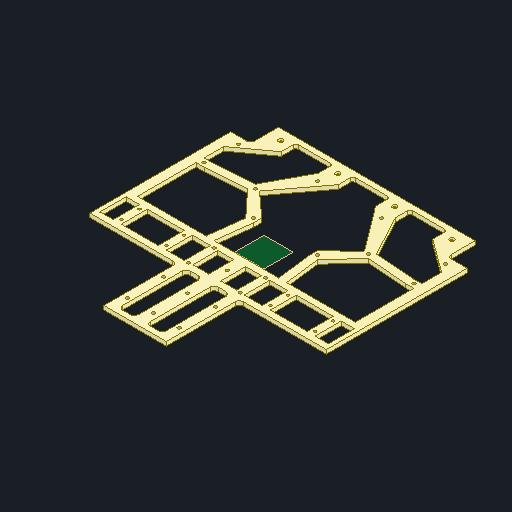
# Autodesk Inventor part: base
Saved by Autodesk Inventor 2023 (Build 270158000, 158)
## iProperties
Created: 2024-04-10
Part Number: base
Material: Nylon 6/6
Document SubType Name: Modeling
Designer: szymo
Density: 1.13 g/cm^3
Appearance: Nylon 6
Mass: 28.9572 g
Surface Area: 254.405 cm^2
Volume: 25.6258 cm^3
Author: szymo
Autodesk Inventor part; units mm, degrees
ref_plane "YZ Plane" through (0, 0, 0) normal (1, 0, 0) x (0, 1, 0)
ref_plane "XZ Plane" through (0, 0, 0) normal (0, 1, 0) x (-1, 0, 0)
ref_plane "XY Plane" through (0, 0, 0) normal (0, 0, 1) x (1, 0, 0)
sketch "Sketch2" plane through (0, 0, 0) normal (0, 1, 0) x (-1, 0, 0)
  line L0 (-89, 99) -> (89, 99)
  line L1 (89, 99) -> (89, -99)
  line L2 (89, -99) -> (-89, -99)
  line L3 (-89, -99) -> (-89, 99)
  line L4 (-89, 99) -> (89, -99) construction
  line L5 (89, 99) -> (-89, -99) construction
  line L6 (-89, 99) -> (89, 99)
  line L7 (89, 99) -> (89, -85)
  line L8 (89, -85) -> (-89, -85)
  line L9 (-89, -85) -> (-89, 99)
  line L10 (-4.5, 99) -> (-89, 99)
  line L11 (-89, 99) -> (-89, 42)
  line L12 (-89, 42) -> (-4.5, 42)
  line L13 (-4.5, 42) -> (-4.5, 99)
  line L14 (4.5, 99) -> (89, 99)
  line L15 (89, 99) -> (89, 42)
  line L16 (89, 42) -> (4.5, 42)
  line L17 (4.5, 42) -> (4.5, 99)
  line L18 (22.5, 77.5) -> (22.5, 66.5) projected
  line L19 (16.5, 66.5) -> (16.5, 77.5) projected
  line L20 (-22.5, 66.5) -> (-22.5, 77.5) projected
  line L21 (-16.5, 77.5) -> (-16.5, 66.5) projected
  line L22 (-23.5, 99) -> (-16.5, 99)
  line L23 (-16.5, 99) -> (-16.5, 42)
  line L24 (-16.5, 42) -> (-23.5, 42)
  line L25 (-23.5, 42) -> (-23.5, 99)
  line L26 (16.5, 99) -> (23.5, 99)
  line L27 (23.5, 99) -> (23.5, 42)
  line L28 (23.5, 42) -> (16.5, 42)
  line L29 (16.5, 42) -> (16.5, 99)
  line L30 (-89, 99) -> (89, 99)
  line L31 (89, 99) -> (89, 97)
  line L32 (89, 97) -> (-89, 97)
  line L33 (-89, 97) -> (-89, 99)
  line L34 (89, -85) -> (74, -85)
  line L35 (74, -85) -> (74, -64)
  line L36 (74, -64) -> (89, -64)
  line L37 (89, -64) -> (89, -85)
  line L38 (-89, -85) -> (-74, -85)
  line L39 (-74, -85) -> (-74, -64)
  line L40 (-74, -64) -> (-89, -64)
  line L41 (-89, -64) -> (-89, -85)
  line L42 (16.5, 97) -> (-16.5, 97)
  line L43 (-16.5, 97) -> (-16.5, 93)
  line L44 (-16.5, 93) -> (16.5, 93)
  line L45 (16.5, 93) -> (16.5, 97)
  line L46 (-84.4, -75) -> (-84.4, -71.5) projected
  line L47 (-84.4, -71.5) -> (-87, -71.5) projected
  line L48 (-87, -71.5) -> (-87, -75) projected
  line L49 (-87, -75) -> (-84.4, -75) projected
  line L50 (-79.6, -75) -> (-77, -75) projected
  line L51 (-77, -75) -> (-77, -71.5) projected
  line L52 (-77, -71.5) -> (-79.6, -71.5) projected
  line L53 (-79.6, -71.5) -> (-79.6, -75) projected
  line L54 (-75, -78) -> (-89, -78) projected
  line L55 (-89, -78) -> (-89, -63) projected
  line L56 (-89, -63) -> (-75, -63) projected
  line L57 (-75, -63) -> (-75, -78) projected
  circle A0 centre (-80.45, -67.25) radius 1.25 projected
  point P0 (0, 0)
  point P1 (4.5, 99)
  point P2 (-4.5, 99)
  point P3 (-89, 42)
  point P4 (89, 42)
  point P5 (4.5, 97)
  point P6 (-4.5, 97)
  point P7 (-16.5, 97)
  point P8 (-23.5, 97)
  point P9 (23.5, 97)
  point P10 (16.5, 98)
  point P11 (-4.5, 93)
  point P12 (4.5, 93)
  point P13 (16.5, 93)
  dimension "d8" = 178
  dimension "d9" = 198
  dimension "d10" = 14
  dimension "d11" = 84.5
  dimension "d13" = 84.5
  dimension "d17" = 9
  dimension "d18" = 2
  dimension "d19" = 15
  dimension "d20" = 21
  dimension "d21" = 15
  dimension "d22" = 21
  dimension "d75" = 55
  dimension "d76" = 55
  dimension "d77" = 7
  dimension "d78" = 7
  dimension "d79" = 4
  constraints: 84 end point, 20 parallel, 10 horizontal, 10 perpendicular, 10 point on line, 2 collinear, 2 midpoint, 5 other
  measures "d8" distance of L1.end L2.end
  measures "d9" distance of L0.end L1.end
  measures "d10" distance between parallel lines of L8 L2
  measures "d11" distance of L12.end L11.end
  measures "d13" distance of L15.end L16.end
  measures "d17" distance between parallel lines of L13 L17
  measures "d18" distance of L30.end L31.end
  measures "d19" distance of L35.end L36.end
  measures "d20" distance of L34.end L35.end
  measures "d21" distance of L40.end L39.end
  measures "d22" distance of L39.end L38.end
  measures "d75" distance between parallel lines of L32 L12
  measures "d76" distance between parallel lines of L32 L16
  measures "d77" distance between parallel lines of L23 L25
  measures "d78" distance between parallel lines of L27 L29
  measures "d79" distance of L43.end L42.end
extrude "Extrusion2" add sketch "Sketch2" along normal blind 3 contours L32 L23 L21 L12 L25 | L12 L13 L44 L17 L16 L1 L36 L35 L8 L39 L40 L57 L56 L3 | L32 L13 L44 L23 | L56 L57 L40 L3 | L32 L17 L44 L13 | L32 L29 L44 L17 | L32 L27 L16 L29 L19
fillet "Fillet5" radius 3 12 edges at (-16.5, 1.5, 42) (-4.5, 1.5, 42) (-23.5, 1.5, 42) (16.5, 1.5, 42) (-16.5, 1.5, 93) (-4.5, 1.5, 93) (4.5, 1.5, 93) (16.5, 1.5, 93) (4.5, 1.5, 42) (23.5, 1.5, 42) (74, 1.5, -64) (-74, 1.5, -64)
sketch "Sketch7" plane through (0, 3, 0) normal (0, 1, 0) x (1, 0, 0)
  circle A0 centre (78, 58.6725) radius 1.8 projected
  circle A1 centre (79, 33.8889) radius 1.8 projected
  circle A2 centre (42.4984, 36.1666) radius 1.8 projected
  circle A3 centre (24.1, 64.6) radius 1.6 projected
  circle A4 centre (24.1, 16.4) radius 1.6 projected
  circle A5 centre (-24.1, 16.4) radius 1.6 projected
  circle A6 centre (-24.1, 64.6) radius 1.6 projected
  circle A7 centre (-42.5, 36.1649) radius 1.8 projected
  circle A8 centre (-79, 33.8889) radius 1.8 projected
  circle A9 centre (-78, 58.6725) radius 1.8 projected
  circle A10 centre (19.5, -18.05) radius 1.8 projected
  circle A11 centre (19.5, -37.375) radius 1.8 projected
  circle A12 centre (19.5, -55.8) radius 1.8 projected
  circle A13 centre (19.4231, -83.3077) radius 1.8 projected
  circle A14 centre (0, -83.2) radius 1.8 projected
  circle A15 centre (-19.4231, -83.3077) radius 1.8 projected
  circle A16 centre (-19.5, -55.8) radius 1.8 projected
  circle A17 centre (0, -57.55) radius 1.8 projected
  circle A18 centre (0, -27.625) radius 1.8 projected
  circle A19 centre (-19.5, -37.375) radius 1.8 projected
  circle A20 centre (-19.5, -18.05) radius 1.8 projected
  point P0 (0, 0)
  point P1 (-19.5, -83.2)
  constraints: 20 coincident
hole "Hole3" at (19.4231, 3, 83.3077) at (0, 3, 83.2) at (-19.5, 3, 83.2) at (19.5, 3, 55.8) at (0, 3, 57.55) at (-19.5, 3, 55.8) at (-19.5, 3, 37.375) at (-19.5, 3, 18.05) at (0, 3, 27.625) at (19.5, 3, 37.375) at (19.5, 3, 18.05) at (79, 3, -33.8889) at (78, 3, -58.6725) at (42.4984, 3, -36.1666) at (24.1, 3, -16.4) at (-24.1, 3, -16.4) at (-24.1, 3, -64.6) at (24.1, 3, -64.6) at (-42.5, 3, -36.1649) at (-78, 3, -58.6725) at (-79, 3, -33.8889) direction (0, -1, 0) diameter 2.459 end through all thread size "M3x0.5" class "6H" standard "ISO Metric profile"
sketch "Sketch8" plane through (0, 3, 0) normal (0, 1, 0) x (1, 0, 0)
  circle A0 centre (86, 37.5556) radius 2.3 projected
  line L0 (89, 40.5556) -> (89, -42) projected
  line L1 (89, 40.5556) -> (83, 40.5556) projected
  line L2 (83, 34.5556) -> (87.4, 34.5556) projected
  line L3 (87.4, 34.5556) -> (87.4, 19.4556) projected
  line L4 (87.4, 19.4556) -> (86, 19.4556) projected
  line L5 (86, -36) -> (86, 19.4556) projected
  circle A1 centre (-86, -39) radius 2.3 projected
  circle A2 centre (-86, -16.25) radius 2.3 projected
  line L6 (-86, -13.25) -> (-86, 29.8889) projected
  line L7 (-86, -36) -> (-86, -19.25) projected
  line L8 (-86, 29.8889) -> (-83, 29.8889) projected
  line L9 (-83, 29.8889) -> (-83, 35.8889) projected
  line L10 (-89, 35.8889) -> (-83, 35.8889) projected
  line L11 (-89, 35.8889) -> (-89, -42) projected
  line L12 (-89, -42) -> (-83, -42) projected
  line L13 (-83, -42) -> (-83, -36) projected
  line L14 (-83, -36) -> (-86, -36) projected
  line L15 (-86, -19.25) -> (-83, -19.25) projected
  line L16 (-83, -19.25) -> (-83, -13.25) projected
  line L17 (-83, -13.25) -> (-86, -13.25) projected
  circle A3 centre (-86, 32.8889) radius 2.3 projected
  ellipse E0 centre (-72.9406, -34.421) end of major axis (-70.1906, -34.421) minor radius 2.75 projected
  ellipse E1 centre (-72.9594, -20.7569) end of major axis (-70.2094, -20.7569) minor radius 2.75 projected
  ellipse E2 centre (-39.125, -20.8137) end of major axis (-36.375, -20.8137) minor radius 2.75 projected
  ellipse E3 centre (-39.125, -34.3886) end of major axis (-36.375, -34.3886) minor radius 2.75 projected
  ellipse E4 centre (39.125, -20.8137) end of major axis (36.375, -20.8137) minor radius 2.75 projected
  ellipse E5 centre (39.125, -34.3886) end of major axis (36.375, -34.3886) minor radius 2.75 projected
  ellipse E6 centre (72.9406, -34.421) end of major axis (70.1906, -34.421) minor radius 2.75 projected
  ellipse E7 centre (72.9594, -20.7569) end of major axis (70.2094, -20.7569) minor radius 2.75 projected
  line L18 (89, -42) -> (83, -42) projected
  line L19 (83, 34.5556) -> (83, 40.5556) projected
  circle A4 centre (86, -39) radius 2.3 projected
  line L20 (86, -36) -> (83, -36) projected
  line L21 (83, -36) -> (83, -42) projected
  point P0 (0, 0)
  point P1 (83, 35.8889)
  point P2 (72.95, -34.475)
  point P3 (72.95, -20.775)
  point P4 (39.125, -20.8375)
  point P5 (39.125, -34.4125)
  point P6 (86, -39)
  point P7 (86, -16.25)
  point P8 (-72.95, -20.775)
  point P9 (-72.95, -34.475)
  point P10 (-39.125, -34.4125)
  point P11 (-39.125, -20.8375)
  constraints: 2 coincident, 4 other
hole "Hole4" at (72.95, 3, 34.475) at (72.95, 3, 20.775) at (39.125, 3, 20.8375) at (39.125, 3, 34.4125) at (-72.95, 3, 20.775) at (-72.95, 3, 34.475) at (-39.125, 3, 34.4125) at (-39.125, 3, 20.8375) direction (0, -1, 0) diameter 2.013 end through all thread size "M2.5x0.45" class "6H" standard "ISO Metric profile"
ref_plane "Work Plane1" through (0, 1, 0) normal (0, -1, 0) x (1, 0, 0)
sketch "Sketch13" plane through (0, 0, 0) normal (0, -1, 0) x (1, 0, 0)
  circle A0 centre (21.5, -77) radius 1.2295 projected
  circle A1 centre (-64.5, -77) radius 1.2295 projected
  circle A2 centre (-21.5, -77) radius 1.2295 projected
  circle A3 centre (64.5, -77) radius 1.2295 projected
  line L0 (-72, -79) -> (-72, -70) projected
  line L1 (-72, -70) -> (-57, -70) projected
  line L2 (-57, -70) -> (-57, -79) projected
  arc A4 (-57, -79) -> (-55, -81) centre (-55, -79) ccw projected
  line L3 (-55, -81) -> (-31, -81) projected
  arc A5 (-31, -81) -> (-29, -79) centre (-31, -79) ccw projected
  line L4 (-29, -79) -> (-29, -70) projected
  line L5 (-29, -70) -> (-14, -70) projected
  line L6 (-14, -70) -> (-14, -79) projected
  arc A6 (-14, -79) -> (-12, -81) centre (-12, -79) ccw projected
  line L7 (-12, -81) -> (12, -81) projected
  arc A7 (12, -81) -> (14, -79) centre (12, -79) ccw projected
  line L8 (14, -79) -> (14, -70) projected
  line L9 (14, -70) -> (29, -70) projected
  line L10 (29, -70) -> (29, -79) projected
  arc A8 (29, -79) -> (31, -81) centre (31, -79) ccw projected
  line L11 (31, -81) -> (55, -81) projected
  arc A9 (55, -81) -> (57, -79) centre (55, -79) ccw projected
  line L12 (57, -79) -> (57, -70) projected
  line L13 (57, -70) -> (72, -70) projected
  line L14 (72, -70) -> (72, -79) projected
  arc A10 (72, -79) -> (74, -81) centre (74, -79) ccw projected
  line L15 (74, -81) -> (89, -81) projected
  line L16 (89, -85) -> (89, -81) projected
  line L17 (-89, -85) -> (89, -85) projected
  line L18 (-89, -85) -> (-89, -81) projected
  line L19 (-89, -81) -> (-74, -81) projected
  arc A11 (-74, -81) -> (-72, -79) centre (-74, -79) ccw projected
  point P0 (0, 0)
  constraints: 4 coincident
hole "Hole6" at (64.5, 0, -77) at (21.5, 0, -77) at (-21.5, 0, -77) at (-64.5, 0, -77) direction (0, 1, 0) diameter 3.6 end through all countersink diameter 6.7 countersink angle 90 clearance for "Countersunk Flat Head Screw ISO 2009/7046" size "M3" standard "ISO"
ref_plane "Work Plane2" through (0, 1, 0) normal (0, -1, 0) x (1, 0, 0)
sketch "Sketch14" plane through (0, 0, 0) normal (0, -1, 0) x (1, 0, 0)
  circle A0 centre (-42.5, -36.1649) radius 1.8 projected
  line L0 (-86, -29.8889) -> (-86, 42) projected
  line L1 (-89, 42) -> (-86, 42) projected
  line L2 (-89, 42) -> (-89, 38.75) projected
  line L3 (-89, 38.75) -> (-89, 13.5) projected
  line L4 (-89, 13.5) -> (-89, -81) projected
  line L5 (-89, -81) -> (-83, -81) projected
  line L6 (-83, -81) -> (-83, -75) projected
  line L7 (-83, -75) -> (-73, -75) projected
  line L8 (-73, -75) -> (-73, -53.3451) projected
  line L9 (-73, -53.3451) -> (-67, -53.3451) projected
  line L10 (-67, -53.3451) -> (-67, -42.9318) projected
  line L11 (-76.801, -42.9318) -> (-67, -42.9318) projected
  ellipse E0 centre (-76.799, -27.2986) end of major axis (-76.7969, -11.6653) minor radius 1.851 (-77.5308, -41.6649) -> (-76.801, -42.9318) ccw projected
  line L12 (-46, -41.6649) -> (-77.5308, -41.6649) projected
  line L13 (-46, -39.6649) -> (-46, -41.6649) projected
  line L14 (-39, -39.6649) -> (-46, -39.6649) projected
  line L15 (-39, -32.6649) -> (-39, -39.6649) projected
  line L16 (-46, -32.6649) -> (-39, -32.6649) projected
  line L17 (-46, -29.8889) -> (-46, -32.6649) projected
  line L18 (-46, -29.8889) -> (-52, -29.8889) projected
  line L19 (-52, -34.8889) -> (-52, -29.8889) projected
  line L20 (-75, -34.8889) -> (-52, -34.8889) projected
  line L21 (-75, -34.8889) -> (-75, -29.8889) projected
  line L22 (-86, -29.8889) -> (-75, -29.8889) projected
  circle A1 centre (-83.5, -70.5) radius 1.75 projected
  circle A2 centre (-79, -33.8889) radius 1.8 projected
  circle A3 centre (-78, -58.6725) radius 1.8 projected
  circle A4 centre (78, -58.6725) radius 1.8 projected
  circle A5 centre (79, -33.8889) radius 1.8 projected
  circle A6 centre (80.5, -70.5) radius 1.75 projected
  circle A7 centre (42.4984, -36.1666) radius 1.8 projected
  spline S0 degree 2 poles (89, 38.051) (88.5208, 39.25) (89, 40.449) knots 0 0 0 0.244949 0.244949 0.244949 weights 1 1.090909 1 projected
  line L23 (89, 42) -> (89, 40.449) projected
  line L24 (89, 42) -> (86, 42) projected
  line L25 (86, -14.7889) -> (86, 42) projected
  line L26 (86, -16.7889) -> (86, -14.7889) projected
  line L27 (86, -27.8889) -> (86, -16.7889) projected
  line L28 (86, -29.8889) -> (86, -27.8889) projected
  line L29 (86, -29.8889) -> (46, -29.8889) projected
  line L30 (46, -32.6649) -> (46, -29.8889) projected
  line L31 (39, -32.6649) -> (46, -32.6649) projected
  line L32 (39, -39.6649) -> (39, -32.6649) projected
  line L33 (46, -39.6649) -> (39, -39.6649) projected
  line L34 (46, -41.6649) -> (46, -39.6649) projected
  line L35 (46, -41.6649) -> (77.5308, -41.6649) projected
  ellipse E1 centre (76.799, -27.2986) end of major axis (76.7969, -11.6653) minor radius 1.851 (76.801, -42.9318) -> (77.5308, -41.6649) ccw projected
  line L36 (76.801, -42.9318) -> (67, -42.9318) projected
  line L37 (67, -53.3451) -> (67, -42.9318) projected
  line L38 (73, -53.3451) -> (67, -53.3451) projected
  line L39 (73, -75) -> (73, -53.3451) projected
  line L40 (83, -75) -> (73, -75) projected
  line L41 (83, -81) -> (83, -75) projected
  line L42 (89, -81) -> (83, -81) projected
  line L43 (89, 14.801) -> (89, -81) projected
  spline S1 degree 2 poles (89, 14.801) (88.5208, 16) (89, 17.199) knots 0 0 0 0.244949 0.244949 0.244949 weights 1 1.090909 1 projected
  line L44 (89, 38.051) -> (89, 17.199) projected
  line L45 (27.5, -68) -> (27.5, -13) projected
  line L46 (27.5, -13) -> (-27.5, -13) projected
  line L47 (-27.5, -13) -> (-27.5, -68) projected
  line L48 (-27.5, -68) -> (27.5, -68) projected
  circle A8 centre (24.1, -64.6) radius 1.6 projected
  circle A9 centre (24.1, -16.4) radius 1.6 projected
  circle A10 centre (-24.1, -64.6) radius 1.6 projected
  circle A11 centre (-24.1, -16.4) radius 1.6 projected
  line L49 (77.6433, -8.75) -> (11.6433, -8.75) projected
  line L50 (77.6433, 11.25) -> (77.6433, -8.75) projected
  line L51 (11.6433, 11.25) -> (77.6433, 11.25) projected
  line L52 (11.6433, -8.75) -> (11.6433, 11.25) projected
  line L53 (-77.0142, -1.75) -> (-9.0142, -1.75) projected
  line L54 (-9.0142, -1.75) -> (-9.0142, 13.25) projected
  line L55 (-9.0142, 13.25) -> (-77.0142, 13.25) projected
  line L56 (-77.0142, 13.25) -> (-77.0142, -1.75) projected
  circle A12 centre (-72.95, 34.475) radius 1.45 projected
  circle A13 centre (-72.95, 20.775) radius 1.45 projected
  circle A14 centre (-39.125, 34.4125) radius 1.55 projected
  circle A15 centre (-39.125, 20.8375) radius 1.55 projected
  line L57 (-27.2, 42) -> (-86, 42) projected
  line L58 (-86, 42) -> (-86, 13.25) projected
  line L59 (-27.2, 13.25) -> (-86, 13.25) projected
  line L60 (-27.2, 13.25) -> (-27.2, 42) projected
  line L61 (27.2, 42) -> (86, 42) projected
  line L62 (27.2, 13.25) -> (27.2, 42) projected
  line L63 (27.2, 13.25) -> (86, 13.25) projected
  line L64 (86, 42) -> (86, 13.25) projected
  line L65 (22.5, 14.25) -> (-22.5, 14.25) projected
  line L66 (-22.5, 14.25) -> (-22.5, 13.25) projected
  line L67 (22.5, 13.25) -> (-22.5, 13.25) projected
  line L68 (22.5, 14.25) -> (22.5, 13.25) projected
  line L69 (-27.2, 13.25) -> (-27.2, 42) projected
  line L70 (-27.2, 13.25) -> (-22.7, 13.25) projected
  line L71 (-22.7, 13.25) -> (-22.7, 42) projected
  line L72 (-27.2, 42) -> (-22.7, 42) projected
  line L73 (27.2, 13.25) -> (27.2, 42) projected
  line L74 (27.2, 42) -> (22.7, 42) projected
  line L75 (22.7, 13.25) -> (22.7, 42) projected
  line L76 (27.2, 13.25) -> (22.7, 13.25) projected
  circle A16 centre (21.5, -77) radius 1.2295 projected
  circle A17 centre (-64.5, -77) radius 1.2295 projected
  circle A18 centre (-21.5, -77) radius 1.2295 projected
  circle A19 centre (64.5, -77) radius 1.2295 projected
  line L77 (-72, -70) -> (-72, -79) projected
  arc A20 (-74, -81) -> (-72, -79) centre (-74, -79) ccw projected
  line L78 (-74, -81) -> (-89, -81) projected
  line L79 (-89, -81) -> (-89, -85) projected
  line L80 (-89, -85) -> (89, -85) projected
  line L81 (89, -81) -> (89, -85) projected
  line L82 (89, -81) -> (74, -81) projected
  arc A21 (72, -79) -> (74, -81) centre (74, -79) ccw projected
  line L83 (72, -79) -> (72, -70) projected
  line L84 (57, -70) -> (72, -70) projected
  line L85 (57, -70) -> (57, -79) projected
  arc A22 (55, -81) -> (57, -79) centre (55, -79) ccw projected
  line L86 (55, -81) -> (31, -81) projected
  arc A23 (29, -79) -> (31, -81) centre (31, -79) ccw projected
  line L87 (29, -79) -> (29, -70) projected
  line L88 (14, -70) -> (29, -70) projected
  line L89 (14, -70) -> (14, -79) projected
  arc A24 (12, -81) -> (14, -79) centre (12, -79) ccw projected
  line L90 (12, -81) -> (-12, -81) projected
  arc A25 (-14, -79) -> (-12, -81) centre (-12, -79) ccw projected
  line L91 (-14, -79) -> (-14, -70) projected
  line L92 (-29, -70) -> (-14, -70) projected
  line L93 (-29, -70) -> (-29, -79) projected
  arc A26 (-31, -81) -> (-29, -79) centre (-31, -79) ccw projected
  line L94 (-31, -81) -> (-55, -81) projected
  arc A27 (-57, -79) -> (-55, -81) centre (-55, -79) ccw projected
  line L95 (-57, -79) -> (-57, -70) projected
  line L96 (-72, -70) -> (-57, -70) projected
  line L97 (-89, -85) -> (-89, -99) projected
  line L98 (-89, -99) -> (89, -99) projected
  line L99 (89, -85) -> (89, -99) projected
  line L100 (-89, -85) -> (89, -85) projected
  circle A28 centre (-21.5, -77) radius 3.35 projected
  circle A29 centre (64.5, -77) radius 3.35 projected
  circle A30 centre (21.5, -77) radius 3.35 projected
  circle A31 centre (-64.5, -77) radius 3.35 projected
  circle A32 centre (-39.125, 34.4125) radius 1.0065 projected
  circle A33 centre (-72.95, 20.775) radius 1.0065 projected
  circle A34 centre (39.125, 20.8375) radius 1.0065 projected
  circle A35 centre (72.95, 34.475) radius 1.0065 projected
  circle A36 centre (72.95, 20.775) radius 1.0065 projected
  circle A37 centre (39.125, 34.4125) radius 1.0065 projected
  circle A38 centre (-72.95, 34.475) radius 1.0065 projected
  circle A39 centre (-39.125, 20.8375) radius 1.0065 projected
  circle A40 centre (-78, -58.6725) radius 1.2295 projected
  circle A41 centre (42.4984, -36.1666) radius 1.2295 projected
  circle A42 centre (79, -33.8889) radius 1.2295 projected
  circle A43 centre (19.5, 37.375) radius 1.2295 projected
  circle A44 centre (-19.5, 18.05) radius 1.2295 projected
  circle A45 centre (-19.5, 55.8) radius 1.2295 projected
  circle A46 centre (19.5, 55.8) radius 1.2295 projected
  circle A47 centre (0, 83.2) radius 1.2295 projected
  circle A48 centre (19.4231, 83.3077) radius 1.2295 projected
  circle A49 centre (-19.5, 83.2) radius 1.2295 projected
  circle A50 centre (0, 57.55) radius 1.2295 projected
  circle A51 centre (-19.5, 37.375) radius 1.2295 projected
  circle A52 centre (0, 27.625) radius 1.2295 projected
  circle A53 centre (19.5, 18.05) radius 1.2295 projected
  circle A54 centre (78, -58.6725) radius 1.2295 projected
  circle A55 centre (-42.5, -36.1649) radius 1.2295 projected
  circle A56 centre (-79, -33.8889) radius 1.2295 projected
  arc A57 (16.5, 90) -> (13.5, 93) centre (13.5, 90) ccw projected
  line L101 (16.5, 45) -> (16.5, 90) projected
  arc A58 (13.5, 42) -> (16.5, 45) centre (13.5, 45) ccw projected
  line L102 (7.5, 42) -> (13.5, 42) projected
  arc A59 (4.5, 45) -> (7.5, 42) centre (7.5, 45) ccw projected
  line L103 (4.5, 90) -> (4.5, 45) projected
  arc A60 (7.5, 93) -> (4.5, 90) centre (7.5, 90) ccw projected
  line L104 (13.5, 93) -> (7.5, 93) projected
  arc A61 (-7.5, 42) -> (-4.5, 45) centre (-7.5, 45) ccw projected
  line L105 (-13.5, 42) -> (-7.5, 42) projected
  arc A62 (-16.5, 45) -> (-13.5, 42) centre (-13.5, 45) ccw projected
  line L106 (-16.5, 90) -> (-16.5, 45) projected
  arc A63 (-13.5, 93) -> (-16.5, 90) centre (-13.5, 90) ccw projected
  line L107 (-7.5, 93) -> (-13.5, 93) projected
  arc A64 (-4.5, 90) -> (-7.5, 93) centre (-7.5, 90) ccw projected
  line L108 (-4.5, 45) -> (-4.5, 90) projected
  arc A65 (-26.5, 42) -> (-23.5, 45) centre (-26.5, 45) ccw projected
  line L109 (-89, 42) -> (-26.5, 42) projected
  line L110 (-89, -64) -> (-89, 42) projected
  line L111 (-77, -64) -> (-89, -64) projected
  arc A66 (-74, -67) -> (-77, -64) centre (-77, -67) ccw projected
  line L112 (-74, -85) -> (-74, -67) projected
  line L113 (74, -85) -> (-74, -85) projected
  line L114 (74, -67) -> (74, -85) projected
  arc A67 (77, -64) -> (74, -67) centre (77, -67) ccw projected
  line L115 (89, -64) -> (77, -64) projected
  line L116 (89, 42) -> (89, -64) projected
  line L117 (26.5, 42) -> (89, 42) projected
  arc A68 (23.5, 45) -> (26.5, 42) centre (26.5, 45) ccw projected
  line L118 (23.5, 97) -> (23.5, 45) projected
  line L119 (-23.5, 97) -> (23.5, 97) projected
  line L120 (-23.5, 45) -> (-23.5, 97) projected
  line L121 (-89, -64) -> (-82, -64)
  line L122 (-82, -64) -> (-82, 42)
  line L123 (-82, 42) -> (-89, 42)
  line L124 (-89, 42) -> (-89, -64)
  line L125 (89, 42) -> (82, 42)
  line L126 (82, 42) -> (82, -64)
  line L127 (82, -64) -> (89, -64)
  line L128 (89, -64) -> (89, 42)
  line L129 (-57, -70) -> (-82, -51.7553)
  line L130 (57, -70) -> (82, -51.7553)
  line L131 (-82, -36.8889) -> (-82, -30.8889)
  line L132 (-82, -30.8889) -> (-76, -30.8889)
  line L133 (-76, -30.8889) -> (-76, -36.8889)
  line L134 (-76, -36.8889) -> (-82, -36.8889)
  line L135 (-82, -36.8889) -> (-76, -30.8889) construction
  line L136 (-82, -30.8889) -> (-76, -36.8889) construction
  line L137 (82, -36.8889) -> (82, -30.8889)
  line L138 (82, -30.8889) -> (76, -30.8889)
  line L139 (76, -30.8889) -> (76, -36.8889)
  line L140 (76, -36.8889) -> (82, -36.8889)
  line L141 (82, -36.8889) -> (76, -30.8889) construction
  line L142 (82, -30.8889) -> (76, -36.8889) construction
  line L143 (-45.5, -39.1649) -> (-39.5, -39.1649)
  line L144 (-39.5, -39.1649) -> (-39.5, -33.1649)
  line L145 (-39.5, -33.1649) -> (-45.5, -33.1649)
  line L146 (-45.5, -33.1649) -> (-45.5, -39.1649)
  line L147 (-45.5, -39.1649) -> (-39.5, -33.1649) construction
  line L148 (-39.5, -39.1649) -> (-45.5, -33.1649) construction
  line L149 (39.4984, -39.1666) -> (39.4984, -33.1666)
  line L150 (39.4984, -33.1666) -> (45.4984, -33.1666)
  line L151 (45.4984, -33.1666) -> (45.4984, -39.1666)
  line L152 (45.4984, -39.1666) -> (39.4984, -39.1666)
  line L153 (39.4984, -39.1666) -> (45.4984, -33.1666) construction
  line L154 (39.4984, -33.1666) -> (45.4984, -39.1666) construction
  line L155 (-76, -30.8889) -> (-45.5, -33.1649)
  line L156 (-76, -36.8889) -> (-45.5, -39.1649)
  line L157 (76, -36.8889) -> (45.4984, -39.1666)
  line L158 (76, -30.8889) -> (45.4984, -33.1666)
  line L159 (-27.1, -19.4) -> (-21.1, -19.4)
  line L160 (-21.1, -19.4) -> (-21.1, -13.4)
  line L161 (-21.1, -13.4) -> (-27.1, -13.4)
  line L162 (-27.1, -13.4) -> (-27.1, -19.4)
  line L163 (-27.1, -19.4) -> (-21.1, -13.4) construction
  line L164 (-21.1, -19.4) -> (-27.1, -13.4) construction
  line L165 (27.1, -19.4) -> (21.1, -19.4)
  line L166 (21.1, -19.4) -> (21.1, -13.4)
  line L167 (21.1, -13.4) -> (27.1, -13.4)
  line L168 (27.1, -13.4) -> (27.1, -19.4)
  line L169 (27.1, -19.4) -> (21.1, -13.4) construction
  line L170 (21.1, -19.4) -> (27.1, -13.4) construction
  line L171 (27.1, -67.6) -> (21.1, -67.6)
  line L172 (21.1, -67.6) -> (21.1, -61.6)
  line L173 (21.1, -61.6) -> (27.1, -61.6)
  line L174 (27.1, -61.6) -> (27.1, -67.6)
  line L175 (27.1, -67.6) -> (21.1, -61.6) construction
  line L176 (21.1, -67.6) -> (27.1, -61.6) construction
  line L177 (-27.1, -67.6) -> (-21.1, -67.6)
  line L178 (-21.1, -67.6) -> (-21.1, -61.6)
  line L179 (-21.1, -61.6) -> (-27.1, -61.6)
  line L180 (-27.1, -61.6) -> (-27.1, -67.6)
  line L181 (-27.1, -67.6) -> (-21.1, -61.6) construction
  line L182 (-21.1, -67.6) -> (-27.1, -61.6) construction
  line L183 (-75.95, 37.475) -> (-69.95, 37.475)
  line L184 (-69.95, 37.475) -> (-69.95, 31.475)
  line L185 (-69.95, 31.475) -> (-75.95, 31.475)
  line L186 (-75.95, 31.475) -> (-75.95, 37.475)
  line L187 (-75.95, 37.475) -> (-69.95, 31.475) construction
  line L188 (-69.95, 37.475) -> (-75.95, 31.475) construction
  line L189 (-75.95, 17.775) -> (-69.95, 17.775)
  line L190 (-69.95, 17.775) -> (-69.95, 23.775)
  line L191 (-69.95, 23.775) -> (-75.95, 23.775)
  line L192 (-75.95, 23.775) -> (-75.95, 17.775)
  line L193 (-75.95, 17.775) -> (-69.95, 23.775) construction
  line L194 (-69.95, 17.775) -> (-75.95, 23.775) construction
  line L195 (-42.125, 23.8375) -> (-36.125, 23.8375)
  line L196 (-36.125, 23.8375) -> (-36.125, 17.8375)
  line L197 (-36.125, 17.8375) -> (-42.125, 17.8375)
  line L198 (-42.125, 17.8375) -> (-42.125, 23.8375)
  line L199 (-42.125, 23.8375) -> (-36.125, 17.8375) construction
  line L200 (-36.125, 23.8375) -> (-42.125, 17.8375) construction
  line L201 (-42.125, 37.4125) -> (-36.125, 37.4125)
  line L202 (-36.125, 37.4125) -> (-36.125, 31.4125)
  line L203 (-36.125, 31.4125) -> (-42.125, 31.4125)
  line L204 (-42.125, 31.4125) -> (-42.125, 37.4125)
  line L205 (-42.125, 37.4125) -> (-36.125, 31.4125) construction
  line L206 (-36.125, 37.4125) -> (-42.125, 31.4125) construction
  line L207 (42.125, 23.8375) -> (36.125, 23.8375)
  line L208 (36.125, 23.8375) -> (36.125, 17.8375)
  line L209 (36.125, 17.8375) -> (42.125, 17.8375)
  line L210 (42.125, 17.8375) -> (42.125, 23.8375)
  line L211 (42.125, 23.8375) -> (36.125, 17.8375) construction
  line L212 (36.125, 23.8375) -> (42.125, 17.8375) construction
  line L213 (42.125, 37.4125) -> (36.125, 37.4125)
  line L214 (36.125, 37.4125) -> (36.125, 31.4125)
  line L215 (36.125, 31.4125) -> (42.125, 31.4125)
  line L216 (42.125, 31.4125) -> (42.125, 37.4125)
  line L217 (42.125, 37.4125) -> (36.125, 31.4125) construction
  line L218 (36.125, 37.4125) -> (42.125, 31.4125) construction
  line L219 (75.95, 37.475) -> (69.95, 37.475)
  line L220 (69.95, 37.475) -> (69.95, 31.475)
  line L221 (69.95, 31.475) -> (75.95, 31.475)
  line L222 (75.95, 31.475) -> (75.95, 37.475)
  line L223 (75.95, 37.475) -> (69.95, 31.475) construction
  line L224 (69.95, 37.475) -> (75.95, 31.475) construction
  line L225 (75.95, 17.775) -> (69.95, 17.775)
  line L226 (69.95, 17.775) -> (69.95, 23.775)
  line L227 (69.95, 23.775) -> (75.95, 23.775)
  line L228 (75.95, 23.775) -> (75.95, 17.775)
  line L229 (75.95, 17.775) -> (69.95, 23.775) construction
  line L230 (69.95, 17.775) -> (75.95, 23.775) construction
  line L231 (-16.5, 37) -> (-4.5, 37)
  line L232 (-4.5, 37) -> (-4.5, 18.25)
  line L233 (-4.5, 18.25) -> (-16.5, 18.25)
  line L234 (-16.5, 18.25) -> (-16.5, 37)
  line L235 (4.5, 37) -> (16.5, 37)
  line L236 (16.5, 37) -> (16.5, 18.25)
  line L237 (16.5, 18.25) -> (4.5, 18.25)
  line L238 (4.5, 18.25) -> (4.5, 37)
  line L239 (-22.5, 40.375) -> (-16.5, 40.375)
  line L240 (-16.5, 40.375) -> (-16.5, 34.375)
  line L241 (-16.5, 34.375) -> (-22.5, 34.375)
  line L242 (-22.5, 34.375) -> (-22.5, 40.375)
  line L243 (-22.5, 40.375) -> (-16.5, 34.375) construction
  line L244 (-16.5, 40.375) -> (-22.5, 34.375) construction
  line L245 (-22.5, 15.05) -> (-16.5, 15.05)
  line L246 (-16.5, 15.05) -> (-16.5, 21.05)
  line L247 (-16.5, 21.05) -> (-22.5, 21.05)
  line L248 (-22.5, 21.05) -> (-22.5, 15.05)
  line L249 (-22.5, 15.05) -> (-16.5, 21.05) construction
  line L250 (-16.5, 15.05) -> (-22.5, 21.05) construction
  line L251 (22.5, 15.05) -> (16.5, 15.05)
  line L252 (16.5, 15.05) -> (16.5, 21.05)
  line L253 (16.5, 21.05) -> (22.5, 21.05)
  line L254 (22.5, 21.05) -> (22.5, 15.05)
  line L255 (22.5, 15.05) -> (16.5, 21.05) construction
  line L256 (16.5, 15.05) -> (22.5, 21.05) construction
  line L257 (22.5, 40.375) -> (16.5, 40.375)
  line L258 (16.5, 40.375) -> (16.5, 34.375)
  line L259 (16.5, 34.375) -> (22.5, 34.375)
  line L260 (22.5, 34.375) -> (22.5, 40.375)
  line L261 (22.5, 40.375) -> (16.5, 34.375) construction
  line L262 (16.5, 40.375) -> (22.5, 34.375) construction
  circle A69 centre (0, 57.55) radius 1.8 projected
  circle A70 centre (0, 27.625) radius 1.8 projected
  circle A71 centre (0, 83.2) radius 1.8 projected
  line L263 (-4.5, 14.25) -> (-4.5, 97) projected
  line L264 (4.5, 14.25) -> (-4.5, 14.25) projected
  line L265 (4.5, 97) -> (4.5, 14.25) projected
  line L266 (-4.5, 97) -> (4.5, 97) projected
  line L267 (-69.95, 37.475) -> (-42.125, 37.475)
  line L268 (-42.125, 37.475) -> (-42.125, 17.8375)
  line L269 (-42.125, 17.8375) -> (-69.95, 17.8375)
  line L270 (-69.95, 17.8375) -> (-69.95, 37.475)
  line L271 (42.125, 37.4125) -> (69.95, 37.4125)
  line L272 (69.95, 37.4125) -> (69.95, 17.775)
  line L273 (69.95, 17.775) -> (42.125, 17.775)
  line L274 (42.125, 17.775) -> (42.125, 37.4125)
  line L275 (-22.5, 14.25) -> (-22.7, 14.25)
  line L276 (-22.5, 13.25) -> (-22.7, 13.25)
  line L277 (22.5, 13.25) -> (24.3333, 13.25)
  line L278 (22.5, 14.25) -> (22.7, 14.25)
  line L279 (45.4984, -39.1666) -> (29, -70)
  line L280 (-29, -70) -> (-45.5, -39.1649)
  line L281 (-14, -70) -> (-39.5, -36.1649)
  line L282 (14, -70) -> (39.4984, -36.1666)
  line L283 (39.4984, -36.1666) -> (21.1, -19.4)
  line L284 (45.4984, -33.1666) -> (27.1, -13.4)
  line L285 (-45.5, -33.1649) -> (-27.1, -13.4)
  line L286 (-39.5, -36.1649) -> (-21.1, -19.4)
  line L287 (27.1, -13.4) -> (30.3333, 13.25)
  line L288 (21.1, -13.4) -> (24.3333, 13.25)
  line L289 (24.1, -13.4) -> (27.3333, 13.25) construction
  line L290 (-24.1, -13.4) -> (-27.3333, 13.25) construction
  line L291 (-21.1, -13.4) -> (-24.3333, 13.25)
  line L292 (-27.1, -13.4) -> (-30.3333, 13.25)
  ellipse E2 centre (72.9406, 34.4114) end of major axis (72.9406, 35.8614) minor radius 1.45 projected
  ellipse E3 centre (72.9594, 20.7472) end of major axis (72.9594, 22.1972) minor radius 1.45 projected
  ellipse E4 centre (39.125, 34.3813) end of major axis (39.125, 35.9313) minor radius 1.55 projected
  ellipse E5 centre (39.125, 20.8063) end of major axis (39.125, 22.3563) minor radius 1.55 projected
  line L293 (66.95, 17.775) -> (45.125, 17.775) projected
  arc A72 (42.125, 20.775) -> (45.125, 17.775) centre (45.125, 20.775) ccw projected
  line L294 (42.125, 20.775) -> (42.125, 34.4125) projected
  arc A73 (45.125, 37.4125) -> (42.125, 34.4125) centre (45.125, 34.4125) ccw projected
  line L295 (45.125, 37.4125) -> (66.95, 37.4125) projected
  arc A74 (69.95, 34.4125) -> (66.95, 37.4125) centre (66.95, 34.4125) ccw projected
  line L296 (69.95, 34.4125) -> (69.95, 20.775) projected
  arc A75 (66.95, 17.775) -> (69.95, 20.775) centre (66.95, 20.775) ccw projected
  line L297 (-75.95, 37.475) -> (-86, 37.475)
  line L298 (-86, 37.475) -> (-86, 17.775)
  line L299 (-86, 17.775) -> (-75.95, 17.775)
  line L300 (-75.95, 17.775) -> (-75.95, 37.475)
  line L301 (75.95, 37.475) -> (86, 37.475)
  line L302 (86, 37.475) -> (86, 17.775)
  line L303 (86, 17.775) -> (75.95, 17.775)
  line L304 (75.95, 17.775) -> (75.95, 37.475)
  line L305 (36.125, 37.4125) -> (22.5, 37.4125)
  line L306 (22.5, 37.4125) -> (22.5, 18.05)
  line L307 (22.5, 18.05) -> (36.125, 18.05)
  line L308 (36.125, 18.05) -> (36.125, 37.4125)
  line L309 (-36.125, 37.4125) -> (-22.5, 37.4125)
  line L310 (-22.5, 37.4125) -> (-22.5, 17.775)
  line L311 (-22.5, 17.775) -> (-36.125, 17.775)
  line L312 (-36.125, 17.775) -> (-36.125, 37.4125)
  point P0 (0, 0)
  point P1 (-82, -36.8889)
  point P2 (74, -75)
  point P3 (73, -58.3234)
  point P4 (82, -36.8889)
  point P5 (82, -30.8889)
  point P6 (82, 13.25)
  point P7 (-82, 13.25)
  point P8 (-82, -29.8889)
  point P9 (-75, -30.9635)
  point P10 (-52, -32.6799)
  point P11 (-82, -30.8889)
  point P12 (82, -29.8889)
  point P13 (-73, -58.3234)
  point P14 (-74, -75)
  point P15 (-82, 42)
  point P16 (79, -57.1759)
  point P17 (79, -60.1692)
  point P18 (39, -36.8279)
  point P19 (39, -35.7124)
  point P20 (79, -59.3878)
  point P21 (79, -57.9572)
  point P22 (27.2, 18.05)
  point P23 (27.2, 37.4125)
  dimension "d217" = 7
  dimension "d218" = 7
  dimension "d219" = 2.459
  dimension "d220" = 3.2295
  dimension "d221" = 3.2295
  dimension "d222" = 6
  dimension "d223" = 6
  dimension "d224" = 6
  dimension "d225" = 6
  dimension "d226" = 6
  dimension "d227" = 6
  dimension "d228" = 6
  dimension "d229" = 6
  dimension "d230" = 6
  dimension "d231" = 6
  dimension "d232" = 6
  dimension "d233" = 6
  dimension "d234" = 6
  dimension "d235" = 6
  dimension "d236" = 6
  dimension "d237" = 6
  dimension "d238" = 6
  dimension "d240" = 6
  dimension "d242" = 6
  dimension "d243" = 6
  dimension "d244" = 6
  dimension "d245" = 6
  dimension "d246" = 6
  dimension "d247" = 6
  dimension "d248" = 6
  dimension "d249" = 6
  dimension "d250" = 6
  dimension "d251" = 6
  dimension "d252" = 6
  dimension "d253" = 6
  dimension "d254" = 6
  dimension "d255" = 6
  dimension "d256" = 6
  dimension "d257" = 6
  dimension "d258" = 6
  dimension "d259" = 6
  dimension "d260" = 6
  dimension "d261" = 6
  dimension "d262" = 5
  dimension "d263" = 5
  dimension "d264" = 5
  dimension "d265" = 5
  dimension "d268" = 54.6667
  dimension "d269" = 54.6667
  dimension "d270" = 54.6667
  dimension "d272" = 6
  dimension "d273" = 6
  constraints: 368 end point, 71 parallel, 37 midpoint, 31 perpendicular, 24 horizontal, 18 point on line, 4 collinear, 6 other
  measures "d217" distance of L123.end L122.end
  measures "d218" distance of L127.end L126.end
  measures "d219" diameter of A40
  measures "d220" distance from line of L129 A40.centre
  measures "d221" distance from line of A4.centre L130
  measures "d222" distance of L131.start L131.end
  measures "d223" distance of L131.end L132.end
  measures "d224" distance of L137.start L137.end
  measures "d225" distance of L138.end L137.end
  measures "d226" distance of L143.start L143.end
  measures "d227" distance of L144.end L143.end
  measures "d228" distance of L149.start L149.end
  measures "d229" distance of L149.end L150.end
  measures "d230" distance of L159.start L159.end
  measures "d231" distance of L160.end L159.end
  measures "d232" distance of L165.start L165.end
  measures "d233" distance of L165.end L166.end
  measures "d234" distance of L171.start L171.end
  measures "d235" distance of L171.end L172.end
  measures "d236" distance of L177.start L177.end
  measures "d237" distance of L178.end L177.end
  measures "d238" distance of L184.end L185.end
  measures "d240" distance of L191.end L190.end
  measures "d242" distance of L196.end L197.end
  measures "d243" distance of L195.end L196.end
  measures "d244" distance of L202.end L203.end
  measures "d245" distance of L201.end L202.end
  measures "d246" distance of L209.end L208.end
  measures "d247" distance of L208.end L207.end
  measures "d248" distance of L215.end L214.end
  measures "d249" distance of L214.end L213.end
  measures "d250" distance of L221.end L220.end
  measures "d251" distance of L220.end L219.end
  measures "d252" distance of L226.end L227.end
  measures "d253" distance of L225.end L226.end
  measures "d254" distance of L240.end L241.end
  measures "d255" distance of L239.end L240.end
  measures "d256" distance of L247.end L246.end
  measures "d257" distance of L246.end L245.end
  measures "d258" distance of L252.end L253.end
  measures "d259" distance of L251.end L252.end
  measures "d260" distance of L259.end L258.end
  measures "d261" distance of L258.end L257.end
  measures "d262" distance between parallel lines of L102 L235
  measures "d263" distance between parallel lines of L67 L237
  measures "d264" distance between parallel lines of L67 L233
  measures "d265" distance between parallel lines of L231 L105
  measures "d268" distance from line of L289.end L126
  measures "d269" distance from line of L290.end L122
  measures "d270" distance of L289.end L290.end
  measures "d272" distance of L185.end L183.start
  measures "d273" distance of L191.end L189.start
extrude "Extrusion7" cut sketch "Sketch14" against normal up to next contours L122 L59 L56 L53 L292 L46 L47 L285 L16 L17 L18 L19 L155 L21 L22 | L22 L21 L155 L132 L122 | L0 L297 L122 L299 | L122 L297 L186 L300 L192 L299 | L55 L292 L53 L56 | L134 L156 L280 L14 L13 L12 E0 L11 L10 L9 L8 L129 L122 | L19 L18 L17 L16 L285 L155 | L111 A66 L112 L7 L6 L5 L4 | L8 L9 L10 L11 E0 L12 L13 L14 L280 L93 A26 L94 A27 L95 L129 | L267 L268 L204 L198 L269 L190 L270 L184 | L55 L54 L53 L291 | L311 L312 L196 L202 L309 L60 | L60 L309 L71 L311 | L53 L54 L67 L277 L76 L288 L51 L52 L49 L46 L291 | L292 L285 L47 L46 | L71 L309 L242 L310 L248 L311 | L46 L288 L166 L283 L45 L282 L48 L281 L47 L286 L160 L291 | L286 L15 L281 | L15 L286 L47 L281 | L281 L48 L282 L89 A24 L90 A25 L91 | L287 L49 L50 L51 L63 L126 L29 L30 L31 L284 L45 L46 | L46 L45 L284 L287 | L49 L52 L51 L288 | L234 L231 L232 L233 | L287 L51 L50 L49 | L283 L32 L282 L45 | L114 L40 L41 L82 | L238 L235 L236 L237 | L307 L254 L306 L260 L305 L75 | L75 L305 L62 L307 | L31 L30 L29 L126 L138 L158 L284 | L42 L41 L40 L114 A67 L115 L43 | L279 L33 L34 L35 E1 L36 L37 L38 L39 L130 L85 A22 L86 A23 L87 | L62 L305 L214 L308 L208 L307 | L279 L157 L140 L126 L130 L39 L38 L37 L36 E1 L35 L34 L33 | L303 L228 L304 L222 L301 L126 | L126 L301 L25 L303 | L271 A73 L216 | L274 L216 A73 L271 A74 L220 L272 L226 A75 L273 A72 L210 | L210 A72 L273 L274 | L273 A75 L226 | L271 L220 A74 | A1 | A6 | A40 | A54
equation "\"d11\" = d13"
body "Solid2"
